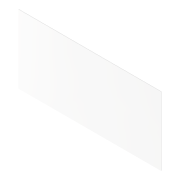
# Autodesk Inventor part: 00_Coverglass_50x24mm
Saved by Autodesk Inventor 2022 (Build 260153000, 153)
## iProperties
Created: 2022-12-18
Part Number: 00_Coverglass_50x24mm
Material: Generisch
Document SubType Name: Modeling
Designer: diederichbenedict
Density: 1 g/cm^3
Appearance: Polycarbonat - klar
Author: diederichbenedict
Autodesk Inventor part; units mm, degrees
ref_plane "YZ Plane" through (0, 0, 0) normal (1, 0, 0) x (0, 1, 0)
ref_plane "XZ Plane" through (0, 0, 0) normal (0, 1, 0) x (-1, 0, 0)
ref_plane "XY Plane" through (0, 0, 0) normal (0, 0, 1) x (1, 0, 0)
sketch "Skizze1" plane through (0, 0, 0) normal (0, 0, 1) x (1, 0, 0)
  line L0 (25, -12) -> (-25, -12)
  line L1 (-25, -12) -> (-25, 12)
  line L2 (-25, 12) -> (25, 12)
  line L3 (25, 12) -> (25, -12)
  line L4 (25, -12) -> (-25, 12) construction
  line L5 (-25, -12) -> (25, 12) construction
  point P0 (0, 0)
  dimension "d0" = 50
  dimension "d1" = 24
  constraints: 12 end point, 2 midpoint, 2 parallel, 1 horizontal, 1 perpendicular
  measures "d0" distance of L1.end L2.end
  measures "d1" distance of L0.end L1.end
extrude "Extrusion1" add sketch "Skizze1" along normal blind 0.2
ref_plane "Arbeitsebene1" through (0, -12, 0) normal (-1, 0, 0) x (0, 0, 1)
